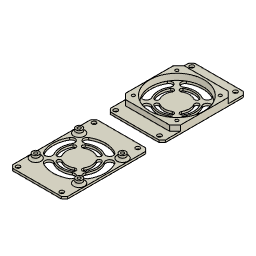
Side Panel - 50mm Fan (Autodesk Fusion 360 design; units mm, degrees)
Autodesk Fusion 360 part; units mm, degrees
ref_plane "WorkPlane2" through (0, 0, 2.999) normal (0, 0, 1) x (1, 0, 0)
sketch "Sketch4" plane through (0, 0, 2.999) normal (0, 0, 1) x (1, 0, 0)
  line L0 (92.5002, -5.0854) -> (92.4954, -5.0854)
  line L1 (89.5002, -5.0854) -> (44.5002, -5.0854) construction
  line L2 (44.5002, -5.0854) -> (41.5002, -8.0854) construction
  line L3 (41.5002, -8.0854) -> (41.5002, -80.0854) construction
  line L4 (41.5002, -80.0854) -> (44.5002, -83.0854) construction
  line L5 (44.5002, -83.0854) -> (89.5002, -83.0854) construction
  line L6 (92.5002, -80.0854) -> (92.5002, -8.0854) construction
  line L7 (86.0002, -79.0854) -> (86.0002, -83.0854) construction
  line L8 (86.0002, -79.0854) -> (92.5002, -79.0854) construction
  line L9 (86.0002, -79.0854) -> (45.705, -79.088) construction
  line L10 (45.7002, -79.0828) -> (41.5002, -79.0831) construction
  line L11 (45.7002, -9.088) -> (45.7002, -5.0854) construction
  line L12 (45.7002, -9.088) -> (45.705, -79.088) construction
  line L13 (45.6956, -9.088) -> (85.9956, -9.0854) construction
  line L14 (85.9956, -9.0854) -> (92.5002, -9.0854) construction
  line L15 (85.9956, -9.0854) -> (85.9956, -5.0854) construction
  line L16 (85.9956, -79.0854) -> (85.9931, -9.0854) construction
  line L17 (92.5002, -80.0854) -> (89.5002, -83.0854) construction
  line L18 (92.5002, -8.0854) -> (89.5002, -5.0854) construction
  line L19 (44.583, -82.8854) -> (89.4174, -82.8854)
  line L20 (92.3002, -80.0026) -> (89.4174, -82.8854)
  line L21 (92.3002, -80.0026) -> (92.3002, -8.1683)
  line L22 (92.3002, -8.1683) -> (89.4174, -5.2854)
  line L23 (89.4174, -5.2854) -> (44.583, -5.2854)
  line L24 (44.583, -5.2854) -> (41.7002, -8.1683)
  line L25 (41.7002, -8.1683) -> (41.7002, -80.0026)
  line L26 (41.7002, -80.0026) -> (44.583, -82.8854)
  circle A0 centre (85.9956, -9.0854) radius 1.9
  circle A1 centre (45.7002, -9.088) radius 1.9
  circle A2 centre (85.9956, -79.0854) radius 1.9
  circle A3 centre (45.7002, -79.0828) radius 1.9
  line L27 (92.5002, -44.0854) -> (41.5002, -44.0854) construction
  point P0 (92.5002, -83.0854)
  point P1 (92.5002, -5.0854)
  dimension "d34" = 6.5
  dimension "d35" = 4
  dimension "d36" = 4.2
  dimension "d37" = 40.2952
  dimension "d38" = 4
  dimension "d39" = 3
  dimension "d40" = 3
  dimension "d43" = 78
  dimension "d44" = 3
  dimension "d45" = 3
  dimension "d46" = 3
  dimension "d47" = 3
  dimension "d48" = 3
  dimension "d49" = 3
  dimension "d50" = -0.2
  dimension "d53" = 3.8
  dimension "d54" = 3.8
  dimension "d55" = 3.8
  dimension "d56" = 3.8
  dimension "d57" = 51
  constraint coincident L5 L7.end
  constraint perpendicular L5 L7
  constraint coincident L6 L8.end
  constraint perpendicular L6 L8
  constraint coincident L3 L10.end
  constraint coincident L1 L11.end
  constraint perpendicular L1 L11
  constraint perpendicular L10 L12
  constraint coincident L6 L14.end
  constraint perpendicular L6 L14
  constraint coincident L1 L15.end
  constraint perpendicular L1 L15
  constraint horizontal L1
  constraint vertical L6
  constraint horizontal L5
  constraint vertical L3
  constraint coincident P0 L6
  constraint coincident P0 L5
  constraint coincident L6 P1
  constraint coincident L1 P1
  constraint coincident L0.start L6
  constraint coincident L0.end L1
  constraint coincident L13.end L14.start
  constraint coincident L11.start L12.start
  constraint coincident L16.start A2.centre
  constraint coincident L10.start A3.centre
  constraint midpoint L6 L27.start
  constraint midpoint L3 L27.end
  constraint symmetric A1 A3 L27
  constraint symmetric A0 A2 L27
  measures "d34" horizontal distance of L7.start L8.end
  measures "d35" vertical distance of L7.start L7.end
  measures "d36" horizontal distance of L10.start L10.end
  measures "d37" horizontal distance of L7.start L9.end
  measures "d38" vertical distance of L13.end L15.end
  measures "d39" horizontal distance of L1.end L2.end
  measures "d40" vertical distance of L1.end L2.end
  measures "d43" distance of L1 L5
  measures "d44" horizontal distance of L3.end L4.end
  measures "d45" vertical distance of L3.end L4.end
  measures "d46" distance of P0 L6.start
  measures "d47" distance of P0 L5.end
  measures "d48" distance of L6.end P1
  measures "d49" distance of L1.start P1
  measures "d53" diameter of A0
  measures "d54" diameter of A1
  measures "d55" diameter of A2
  measures "d56" diameter of A3
  measures "d57" distance of L3 L6
extrude "Extrude11" add sketch "Sketch4" against normal blind 2 makes body 1
sketch "Sketch5" plane through (0, 0, 2.999) normal (0, 0, 1) x (-1, 0, 0)
  circle A0 centre (-85.9956, 9.0854) radius 1.9
  circle A1 centre (-45.7002, 79.0828) radius 1.9
  circle A2 centre (-85.9956, 79.0854) radius 1.9
  circle A3 centre (-45.7002, 9.088) radius 1.9
  line L0 (-92.3002, 80.0026) -> (-92.3002, 8.1683)
  line L1 (-92.3002, 8.1683) -> (-89.4174, 5.2854)
  line L2 (-89.4174, 5.2854) -> (-44.583, 5.2854)
  line L3 (-44.583, 5.2854) -> (-41.7002, 8.1683)
  line L4 (-41.7002, 8.1683) -> (-41.7002, 80.0026)
  line L5 (-41.7002, 80.0026) -> (-44.583, 82.8854)
  line L6 (-44.583, 82.8854) -> (-89.4174, 82.8854)
  line L7 (-89.4174, 82.8854) -> (-92.3002, 80.0026)
  line L8 (-43.1416, 6.7268) -> (-90.8588, 81.444) construction
  line L9 (-90.8588, 6.7268) -> (-43.1416, 81.444) construction
  circle A4 centre (-67.0002, 44.0854) radius 24
  line L10 (-87.0002, 64.0854) -> (-47.0002, 64.0854) construction
  line L11 (-47.0002, 64.0854) -> (-47.0002, 24.0854) construction
  line L12 (-47.0002, 24.0854) -> (-87.0002, 24.0854) construction
  line L13 (-87.0002, 24.0854) -> (-87.0002, 64.0854) construction
  line L14 (-87.0002, 64.0854) -> (-47.0002, 24.0854) construction
  line L15 (-47.0002, 64.0854) -> (-87.0002, 24.0854) construction
  circle A5 centre (-87.0002, 24.0854) radius 1.4
  circle A6 centre (-87.0002, 64.0854) radius 1.4
  circle A7 centre (-47.0002, 64.0854) radius 1.4
  circle A8 centre (-47.0002, 24.0854) radius 1.4
  circle A9 centre (-47.0002, 64.0854) radius 3
  circle A10 centre (-87.0002, 64.0854) radius 3
  circle A11 centre (-87.0002, 24.0854) radius 3
  circle A12 centre (-47.0002, 24.0854) radius 3
  point P0 (-67.0002, 44.0854)
  dimension "d58" = 48
  dimension "d59" = 40
  dimension "d60" = 40
  dimension "d61" = 2.8
  dimension "d62" = 2.8
  dimension "d63" = 2.8
  dimension "d64" = 2.8
  dimension "d77" = 1.6
  dimension "d78" = 1.6
  dimension "d79" = 1.6
  dimension "d80" = 1.6
  constraint midpoint L3 L8.start
  constraint midpoint L7 L8.end
  constraint midpoint L1 L9.start
  constraint midpoint L5 L9.end
  constraint midpoint L8 P0
  constraint horizontal L10
  constraint perpendicular L10 L11
  constraint parallel L10 L12
  constraint parallel L11 L13
  constraint coincident L14 P0
  constraint coincident L15 P0
  constraint coincident P0 A4.centre
  constraint coincident L12.end L13.start
  constraint coincident L10.start L13.end
  constraint coincident L10.end L11.start
  constraint coincident L11.end L12.start
  measures "d58" diameter of A4
  measures "d59" distance of L11.end L12.end
  measures "d60" distance of L10.end L11.end
  measures "d61" diameter of A5
  measures "d62" diameter of A6
  measures "d63" diameter of A7
  measures "d64" diameter of A8
extrude "Extrude12" cut sketch "Sketch5" against normal blind 2 contours A4 | A5 | A6 | A7 | A8 bodies 1
copy_body "Body->Comp2" bodies 1 removing the originals makes body 2 in component "Side Panel - External 50mm Fan"
copy_body "CopyPasteBodies1" bodies 2 makes body 3 in component "Side Panel - Internal 50mm Fan"
move_body "Move1" bodies 3 to x (1, 0, 0) y (0, 1, 0) z (0, 0, 1) at (0, 0, 0) in component "Side Panel - Internal 50mm Fan"
sketch "Sketch1" plane through (0, 0, 2.999) normal (0, 0, 1) x (-1, 0, 0) in component "Side Panel - Internal 50mm Fan"
  circle A0 centre (-87.0002, 24.0854) radius 1.4
  circle A1 centre (-47.0002, 24.0854) radius 1.4
  circle A2 centre (-87.0002, 64.0854) radius 1.4
  circle A3 centre (-67.0002, 44.0854) radius 24
  circle A4 centre (-47.0002, 64.0854) radius 1.4
  circle A5 centre (-85.9956, 9.0854) radius 1.9
  circle A6 centre (-45.7002, 79.0828) radius 1.9
  circle A7 centre (-85.9956, 79.0854) radius 1.9
  circle A8 centre (-45.7002, 9.088) radius 1.9
  line L0 (-92.3002, 80.0026) -> (-92.3002, 8.1683)
  line L1 (-92.3002, 8.1683) -> (-89.4174, 5.2854)
  line L2 (-89.4174, 5.2854) -> (-44.583, 5.2854)
  line L3 (-44.583, 5.2854) -> (-41.7002, 8.1683)
  line L4 (-41.7002, 8.1683) -> (-41.7002, 80.0026)
  line L5 (-41.7002, 80.0026) -> (-44.583, 82.8854)
  line L6 (-44.583, 82.8854) -> (-89.4174, 82.8854)
  line L7 (-89.4174, 82.8854) -> (-92.3002, 80.0026)
  circle A9 centre (-67.0002, 44.0854) radius 10 construction
  line L8 (-67.0002, 34.0854) -> (-67.0002, 20.0854) construction
  line L9 (-72.0002, 35.4252) -> (-79.0002, 23.3008) construction
  line L10 (-67.0002, 44.0854) -> (-43.0002, 44.0854) construction
  line L11 (-62.0002, 35.4252) -> (-55.0002, 23.3008) construction
  line L12 (-58.5002, 29.363) -> (-62.0002, 35.4252) construction
  line L13 (-72.0002, 35.4252) -> (-75.5002, 29.363) construction
  line L14 (-67.0002, 34.0854) -> (-67.0002, 27.0854) construction
  line L15 (-67.0002, 27.0854) -> (-67.0002, 20.0854) construction
  line L16 (-58.5002, 29.363) -> (-55.0002, 23.3008) construction
  line L17 (-75.5002, 29.363) -> (-79.0002, 23.3008) construction
  arc A10 (-79.0002, 23.3008) -> (-55.0002, 23.3008) centre (-67.0002, 44.0854) ccw
  arc A11 (-75.5002, 29.363) -> (-79.0002, 23.3008) centre (-77.2502, 26.3319) ccw
  arc A12 (-75.5002, 29.363) -> (-58.5002, 29.363) centre (-67.0002, 44.0854) ccw
  arc A13 (-55.0002, 23.3008) -> (-58.5002, 29.363) centre (-56.7502, 26.3319) ccw
  arc A14 (-77.2502, 26.3319) -> (-56.7502, 26.3319) centre (-67.0002, 44.0854) ccw construction
  arc A15 (-74.7502, 30.662) -> (-59.2502, 30.662) centre (-67.0002, 44.0854) ccw
  arc A16 (-72.7502, 34.1261) -> (-74.7502, 30.662) centre (-73.7502, 32.3941) ccw
  arc A17 (-72.7502, 34.1261) -> (-61.2502, 34.1261) centre (-67.0002, 44.0854) ccw
  arc A18 (-59.2502, 30.662) -> (-61.2502, 34.1261) centre (-60.2502, 32.3941) ccw
  arc A19 (-73.7502, 32.3941) -> (-60.2502, 32.3941) centre (-67.0002, 44.0854) ccw construction
  arc A20 (-53.5768, 51.8354) -> (-57.0409, 49.8354) centre (-55.3089, 50.8354) ccw
  arc A21 (-53.5768, 36.3354) -> (-53.5768, 51.8354) centre (-67.0002, 44.0854) ccw
  arc A22 (-57.0409, 38.3354) -> (-53.5768, 36.3354) centre (-55.3089, 37.3354) ccw
  arc A23 (-57.0409, 38.3354) -> (-57.0409, 49.8354) centre (-67.0002, 44.0854) ccw
  arc A24 (-52.2778, 35.5854) -> (-52.2778, 52.5854) centre (-67.0002, 44.0854) ccw
  arc A25 (-52.2778, 35.5854) -> (-46.2156, 32.0854) centre (-49.2467, 33.8354) ccw
  arc A26 (-46.2156, 32.0854) -> (-46.2156, 56.0854) centre (-67.0002, 44.0854) ccw
  arc A27 (-46.2156, 56.0854) -> (-52.2778, 52.5854) centre (-49.2467, 54.3354) ccw
  arc A28 (-74.7502, 57.5088) -> (-72.7502, 54.0447) centre (-73.7502, 55.7768) ccw
  arc A29 (-59.2502, 57.5088) -> (-74.7502, 57.5088) centre (-67.0002, 44.0854) ccw
  arc A30 (-61.2502, 54.0447) -> (-59.2502, 57.5088) centre (-60.2502, 55.7768) ccw
  arc A31 (-61.2502, 54.0447) -> (-72.7502, 54.0447) centre (-67.0002, 44.0854) ccw
  arc A32 (-58.5002, 58.8079) -> (-75.5002, 58.8079) centre (-67.0002, 44.0854) ccw
  arc A33 (-58.5002, 58.8079) -> (-55.0002, 64.87) centre (-56.7502, 61.8389) ccw
  arc A34 (-55.0002, 64.87) -> (-79.0002, 64.87) centre (-67.0002, 44.0854) ccw
  arc A35 (-79.0002, 64.87) -> (-75.5002, 58.8079) centre (-77.2502, 61.8389) ccw
  arc A36 (-80.4236, 36.3354) -> (-76.9595, 38.3354) centre (-78.6915, 37.3354) ccw
  arc A37 (-80.4236, 51.8354) -> (-80.4236, 36.3354) centre (-67.0002, 44.0854) ccw
  arc A38 (-76.9595, 49.8354) -> (-80.4236, 51.8354) centre (-78.6915, 50.8354) ccw
  arc A39 (-76.9595, 49.8354) -> (-76.9595, 38.3354) centre (-67.0002, 44.0854) ccw
  arc A40 (-81.7226, 52.5854) -> (-81.7226, 35.5854) centre (-67.0002, 44.0854) ccw
  arc A41 (-81.7226, 52.5854) -> (-87.7848, 56.0854) centre (-84.7537, 54.3354) ccw
  arc A42 (-87.7848, 56.0854) -> (-87.7848, 32.0854) centre (-67.0002, 44.0854) ccw
  arc A43 (-87.7848, 32.0854) -> (-81.7226, 35.5854) centre (-84.7537, 33.8354) ccw
  dimension "d67" = 20
  dimension "d68" = 120
  dimension "d69" = 7
  dimension "d70" = 4
  dimension "d72" = 360
  constraint concentric A3 A9
  constraint coincident A3.centre A9.centre
  constraint coincident A3 L8.end
  constraint vertical L8
  constraint horizontal L10
  constraint coincident A9 L9.start
  constraint symmetric L8 L9.end L11.end
  constraint symmetric L8 L9.start L11.start
  constraint coincident A9 L8.start
  constraint midpoint L11 L12.start
  constraint parallel L11 L12
  constraint midpoint L9 L13.end
  constraint midpoint L8 L14.end
  constraint parallel L9 L17
  constraint tangent A10 A11
  constraint tangent A11 A12
  constraint tangent A12 A13
  constraint tangent A10 A13
  constraint midpoint L17 A11.centre
  constraint midpoint L16 A13.centre
  constraint tangent A15 A16
  constraint tangent A16 A17
  constraint tangent A17 A18
  constraint tangent A15 A18
  constraint midpoint L13 A16.centre
  constraint midpoint L12 A18.centre
  measures "d67" diameter of A9
  measures "d68" angle of L9 L10
  measures "d69" diameter of A13
  measures "d70" diameter of A18
extrude "Extrude1" add sketch "Sketch1" against normal blind 2 contours A3 A11 A12 A13 A24 A25 A27 A32 A33 A35 A40 A41 A43 bodies 3 in component "Side Panel - Internal 50mm Fan"
sketch "Sketch2" plane through (0, 0, 2.999) normal (0, 0, 1) x (-1, 0, 0) in component "Side Panel - Internal 50mm Fan"
  circle A0 centre (-87.0002, 24.0854) radius 1.4
  circle A1 centre (-47.0002, 24.0854) radius 1.4
  circle A2 centre (-87.0002, 64.0854) radius 1.4
  circle A3 centre (-67.0002, 44.0854) radius 24
  circle A4 centre (-47.0002, 64.0854) radius 1.4
  circle A5 centre (-85.9956, 9.0854) radius 1.9
  circle A6 centre (-45.7002, 79.0828) radius 1.9
  circle A7 centre (-85.9956, 79.0854) radius 1.9
  circle A8 centre (-45.7002, 9.088) radius 1.9
  line L0 (-92.3002, 80.0026) -> (-92.3002, 8.1683)
  line L1 (-92.3002, 8.1683) -> (-89.4174, 5.2854)
  line L2 (-89.4174, 5.2854) -> (-44.583, 5.2854)
  line L3 (-44.583, 5.2854) -> (-41.7002, 8.1683)
  line L4 (-41.7002, 8.1683) -> (-41.7002, 80.0026)
  line L5 (-41.7002, 80.0026) -> (-44.583, 82.8854)
  line L6 (-44.583, 82.8854) -> (-89.4174, 82.8854)
  line L7 (-89.4174, 82.8854) -> (-92.3002, 80.0026)
  line L8 (-87.3002, 71.0854) -> (-46.7002, 71.0854)
  line L9 (-41.7002, 66.0854) -> (-41.7002, 22.0854)
  line L10 (-46.7002, 17.0854) -> (-87.3002, 17.0854)
  line L11 (-92.3002, 22.0854) -> (-92.3002, 66.0854)
  line L12 (-92.3002, 71.0854) -> (-41.7002, 17.0854) construction
  line L13 (-41.7002, 71.0854) -> (-92.3002, 17.0854) construction
  line L14 (-46.7002, 71.0854) -> (-41.7002, 66.0854)
  line L15 (-87.3002, 71.0854) -> (-92.3002, 66.0854)
  line L16 (-92.3002, 22.0854) -> (-87.3002, 17.0854)
  line L17 (-46.7002, 17.0854) -> (-41.7002, 22.0854)
  point P0 (-67.0002, 44.0854)
  dimension "d75" = 54
  dimension "d91" = 5
  dimension "d92" = 5
  dimension "d93" = 5
  dimension "d94" = 5
  dimension "d95" = 5
  dimension "d96" = 5
  dimension "d97" = 5
  dimension "d98" = 5
  constraint horizontal L8
  constraint perpendicular L8 L9
  constraint parallel L8 L10
  constraint parallel L9 L11
  constraint coincident L12 P0
  constraint coincident L13 P0
  constraint coincident L0 L12.start
  constraint coincident P0 A3.centre
  constraint coincident L13.start L8
  constraint coincident L13.start L9
  constraint coincident L12.start L8
  constraint coincident L12.start L11
  constraint coincident L13.end L11
  constraint coincident L13.end L10
  constraint coincident L12.end L10
  constraint coincident L12.end L9
  measures "d75" distance of L13.start L12.end
  measures "d91" distance of L13.start L8.end
  measures "d92" distance of L13.start L9.start
  measures "d93" distance of L12.start L8.start
  measures "d94" distance of L12.start L11.end
  measures "d95" distance of L13.end L11.start
  measures "d96" distance of L13.end L10.end
  measures "d97" distance of L12.end L10.start
  measures "d98" distance of L12.end L9.end
extrude "Extrude1'" add sketch "Sketch5" along normal blind 4 contours A9 | A10 | A11 | A12 bodies 2 in component "Side Panel - External 50mm Fan"
extrude "Extrude2" add sketch "Sketch1" against normal blind 2 contours A3 A11 A12 A13 A24 A25 A27 A32 A33 A35 A40 A41 A43 bodies 2 in component "Side Panel - External 50mm Fan"
fillet "Fillet1" radius 2 4 edges at (89.7972, -65.1703, 2.999) (49.7972, -65.1703, 2.999) (49.7972, -25.1703, 2.999) (89.7972, -25.1703, 2.999) on bodies 2 in component "Side Panel - External 50mm Fan"
extrude "Extrude2'" add sketch "Sketch2" against normal blind 2 contours A0 | A1 | A2 | A4 bodies 3 in component "Side Panel - Internal 50mm Fan"
extrude "Extrude3" add sketch "Sketch2" along normal blind 5 contours L0 L4 L8 L9 L10 L11 L14 L15 L16 L17 bodies 3 in component "Side Panel - Internal 50mm Fan"
chamfer "Chamfer1" distance 1 distance2 5 1 edges at (89.3761, -52.7642, 7.999) measured on face at (49.909, -21.1731, 7.999) on bodies 3 in component "Side Panel - Internal 50mm Fan"
component "Side Panel - Internal 50mm Fan" placed x (1, 0, 0) y (0, 1, 0) z (0, 0, 1) at (0, 0, 0)
component "Side Panel - External 50mm Fan" placed x (1, 0, 0) y (0, 1, 0) z (0, 0, 1) at (0, -90, 0)
equation "d39 = d40"
equation "d40 = d44"
equation "d45 = d44"
equation "d46 = d44"
equation "d47 = d46"
equation "d48 = d44"
equation "d49 = d48"
equation "d53 = d55"
equation "d54 = d55"
equation "d56 = d55"
equation "d61 = d63"
equation "d62 = d63"
equation "d64 = d63"
equation "d93 = d91"
equation "d94 = d91"
equation "d95 = d91"
equation "d96 = d91"
equation "d97 = d91"
equation "d98 = d91"
